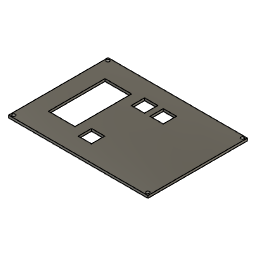
Music Playerr Lid V1 (Autodesk Fusion 360 design; units mm, degrees)
Autodesk Fusion 360 part; units mm, degrees
box "BoxPrimitive1" add length 47.625 width 66.675 height 1.143 placed x (0, -1, 0) y (1, 0, 0) z (0, 0, 1) at (0, 0, 0)
hole "Hole1" at (65.3321, -46.3308, 1.143) direction (0, 0, -1) diameter 2 depth 10.16 tip angle 180
hole "Hole2" at (1.2247, -46.3698, 1.143) direction (0, 0, -1) diameter 2.0066 depth 10.16 tip angle 180
hole "Hole3" at (1.2016, -1.2479, 1.143) direction (0, 0, -1) diameter 2.0066 depth 10.16 tip angle 180
hole "Hole4" at (65.4587, -1.1437, 1.143) direction (0, 0, -1) diameter 2.0066 depth 10.16 tip angle 180
thread "Thread1" "ANSI Unified Screw Threads 0.073(#1) 1-64 UNC 3B" major diameter 1.8542 minor diameter 1.5037 pitch 0.3969 angle 60 resizes the face on face at (65.8018, -2.0865, 0.762)
thread "Thread2" "ANSI Unified Screw Threads 0.073(#1) 1-64 UNC 3B" major diameter 1.8542 minor diameter 1.5037 pitch 0.3969 angle 60 resizes the face on face at (64.9437, -47.2523, 0.762)
thread "Thread3" "ANSI Unified Screw Threads 0.073(#1) 1-64 UNC 3B" major diameter 1.8542 minor diameter 1.5037 pitch 0.3969 angle 60 resizes the face on face at (1.2747, -47.3719, 0.762)
thread "Thread4" "ANSI Unified Screw Threads 0.073(#1) 1-64 UNC 3B" major diameter 1.8542 minor diameter 1.5037 pitch 0.3969 angle 60 resizes the face on face at (1.2516, -2.2499, 0.762)
sketch "Sketch2" plane through (0, 0, 1.143) normal (0, 0, 1) x (-1, 0, 0)
  circle A0 centre (-65.4587, 1.1437) radius 0.7518
  circle A1 centre (-1.2016, 1.2479) radius 0.7518
  circle A2 centre (-1.2247, 46.3698) radius 0.7518
  circle A3 centre (-65.3321, 46.3308) radius 0.7518
  line L0 (0, 47.625) -> (-66.675, 47.625)
  line L1 (-66.675, 47.625) -> (-66.675, 0)
  line L2 (-66.675, 0) -> (0, 0)
  line L3 (0, 0) -> (0, 47.625)
  line L4 (-7.9375, 9.4361) -> (-20.6375, 9.4361)
  line L5 (-20.6375, 9.4361) -> (-20.6375, 36.5014)
  line L6 (-20.6375, 36.5014) -> (-7.9375, 36.5014)
  line L7 (-7.9375, 36.5014) -> (-7.9375, 9.4361)
  line L8 (-25.371, 39.6857) -> (-31.721, 39.6857)
  line L9 (-31.721, 39.6857) -> (-31.721, 33.3262)
  line L10 (-31.721, 33.3262) -> (-25.371, 33.3262)
  line L11 (-25.371, 33.3262) -> (-25.371, 39.6857)
  line L12 (-25.371, 7.927) -> (-25.371, 14.2865)
  line L13 (-31.721, 7.927) -> (-25.371, 7.927)
  line L14 (-25.371, 14.2865) -> (-31.721, 14.2865)
  line L15 (-31.721, 14.2865) -> (-31.721, 7.927)
  line L16 (-34.3146, 14.2865) -> (-40.6646, 14.2865)
  line L17 (-34.3146, 7.927) -> (-34.3146, 14.2865)
  line L18 (-40.6646, 7.927) -> (-34.3146, 7.927)
  line L19 (-40.6646, 14.2865) -> (-40.6646, 7.927)
  dimension "d18" = 12.7
  dimension "d19" = 6.35
  dimension "d20" = 6.35
  dimension "d21" = 6.35
  constraint horizontal L4
  constraint vertical L5
  constraint horizontal L6
  constraint vertical L7
  constraint horizontal L8
  constraint vertical L9
  constraint horizontal L10
  constraint vertical L11
  constraint horizontal L14
  constraint vertical L15
  constraint horizontal L13
  constraint vertical L12
  constraint horizontal L16
  constraint vertical L19
  constraint horizontal L18
  constraint vertical L17
  measures "d18" distance of L4.start L4.end
  measures "d19" distance of L8.start L8.end
  measures "d20" distance of L12.end L14.end
  measures "d21" distance of L16.end L16.start
extrude "Extrude1" cut sketch "Sketch2" against normal blind 87.7062 contours L4 L5 L6 L7 | L8 L9 L10 L11 | L12 L13 L14 L15 | L16 L17 L18 L19
